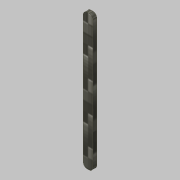
# Autodesk Inventor part: Microphone_hole_plug
Saved by Autodesk Inventor 2019.3 (Build 233278000, 278)
## iProperties
Created: 2019-02-18
Part Number: Microphone_hole_plug
Material: Generic
Document SubType Name: Modeling
Designer: Varga Daniel
Density: 1 g/cm^3
Appearance: Carbon Fiber 1
Author: Varga Daniel
Autodesk Inventor part; units mm, degrees
ref_plane "YZ Plane" through (0, 0, 0) normal (1, 0, 0) x (0, 1, 0)
ref_plane "Work Plane3" through (0, 0, 0) normal (0, 0, 1) x (1, 0, 0)
sketch "Sketch1" plane through (0, 0, 0) normal (0, 0, 1) x (1, 0, 0)
  line L0 (-60, 40) -> (60, 40) projected
  line L1 (-60, -40) -> (-60, 40) projected
  line L2 (-60, -40) -> (60, -40) projected
  line L3 (60, 40) -> (60, -40) projected
  circle A0 centre (-46, -15) radius 2 projected
  circle A1 centre (-46, 15) radius 2 projected
  circle A2 centre (-46, 5) radius 2 projected
  circle A3 centre (-46, -5) radius 2 projected
  circle A4 centre (-3, 0) radius 24 projected
  line L4 (-38.25, 16.5) -> (-38.25, -16.5) projected
  arc A5 (-37.25, 17.5) -> (-38.25, 16.5) centre (-37.25, 16.5) ccw projected
  line L5 (-36.75, 17.5) -> (-37.25, 17.5) projected
  arc A6 (-35.75, 16.5) -> (-36.75, 17.5) centre (-36.75, 16.5) ccw projected
  line L6 (-35.75, -16.5) -> (-35.75, 16.5) projected
  arc A7 (-36.75, -17.5) -> (-35.75, -16.5) centre (-36.75, -16.5) ccw projected
  line L7 (-37.25, -17.5) -> (-36.75, -17.5) projected
  arc A8 (-38.25, -16.5) -> (-37.25, -17.5) centre (-37.25, -16.5) ccw projected
  arc A9 (47, 6.4964) -> (46.6925, 7.2389) centre (45.95, 6.4964) ccw projected
  line L8 (47, 1.3036) -> (47, 6.4964) projected
  arc A10 (46.6925, 0.5611) -> (47, 1.3036) centre (45.95, 1.3036) ccw projected
  line L9 (46.0889, -0.0425) -> (46.6925, 0.5611) projected
  arc A11 (45.3464, -0.35) -> (46.0889, -0.0425) centre (45.3464, 0.7) ccw projected
  line L10 (44.6, -0.35) -> (45.3464, -0.35) projected
  arc A12 (43.55, 0.7) -> (44.6, -0.35) centre (44.6, 0.7) ccw projected
  line L11 (43.55, 7.1) -> (43.55, 0.7) projected
  arc A13 (44.6, 8.15) -> (43.55, 7.1) centre (44.6, 7.1) ccw projected
  line L12 (45.3464, 8.15) -> (44.6, 8.15) projected
  arc A14 (46.0889, 7.8425) -> (45.3464, 8.15) centre (45.3464, 7.1) ccw projected
  line L13 (46.6925, 7.2389) -> (46.0889, 7.8425) projected
  arc A15 (46.0889, 20.4425) -> (45.3464, 20.75) centre (45.3464, 19.7) ccw projected
  line L14 (46.6925, 19.8389) -> (46.0889, 20.4425) projected
  arc A16 (47, 19.0964) -> (46.6925, 19.8389) centre (45.95, 19.0964) ccw projected
  line L15 (47, 13.9036) -> (47, 19.0964) projected
  arc A17 (46.6925, 13.1611) -> (47, 13.9036) centre (45.95, 13.9036) ccw projected
  line L16 (46.0889, 12.5575) -> (46.6925, 13.1611) projected
  arc A18 (45.3464, 12.25) -> (46.0889, 12.5575) centre (45.3464, 13.3) ccw projected
  line L17 (44.6, 12.25) -> (45.3464, 12.25) projected
  arc A19 (43.55, 13.3) -> (44.6, 12.25) centre (44.6, 13.3) ccw projected
  line L18 (43.55, 19.7) -> (43.55, 13.3) projected
  arc A20 (44.6, 20.75) -> (43.55, 19.7) centre (44.6, 19.7) ccw projected
  line L19 (45.3464, 20.75) -> (44.6, 20.75) projected
  arc A21 (44.9066, -31.2) -> (45.7117, -30.824) centre (44.9066, -30.15) ccw projected
  line L20 (43.6, -31.2) -> (44.9066, -31.2) projected
  arc A22 (42.55, -30.15) -> (43.6, -31.2) centre (43.6, -30.15) ccw projected
  line L21 (42.55, -20.05) -> (42.55, -30.15) projected
  arc A23 (43.6, -19) -> (42.55, -20.05) centre (43.6, -20.05) ccw projected
  line L22 (44.9066, -19) -> (43.6, -19) projected
  arc A24 (45.7117, -19.376) -> (44.9066, -19) centre (44.9066, -20.05) ccw projected
  line L23 (46.5051, -20.3236) -> (45.7117, -19.376) projected
  arc A25 (46.75, -20.9977) -> (46.5051, -20.3236) centre (45.7, -20.9977) ccw projected
  line L24 (46.75, -29.2023) -> (46.75, -20.9977) projected
  arc A26 (46.5051, -29.8764) -> (46.75, -29.2023) centre (45.7, -29.2023) ccw projected
  line L25 (45.7117, -30.824) -> (46.5051, -29.8764) projected
  point P0 (0, 0)
ref_plane "Work Plane2" through (-58, -38, -1) normal (0, 0, -1) x (0, 1, 0)
extrude "Extrusion1" add sketch "Sketch1" against normal up to surface (1 mm away) contours A5 L5 A6 L6 A7 L7 A8 L4
body "Solid1"
